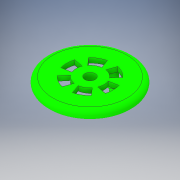
# Autodesk Inventor part: train wheel.
Saved by Autodesk Inventor 2017 (Build 210142000, 142)
## iProperties
Created: 2017-04-27
Part Number: train wheel.
Material: Generic
Document SubType Name: Modeling
Designer: 167898
Density: 1 g/cm^3
Appearance: Default
Author: 167898
Autodesk Inventor part; units mm, degrees
ref_plane "YZ Plane" through (0, 0, 0) normal (1, 0, 0) x (0, 1, 0)
ref_plane "XZ Plane" through (0, 0, 0) normal (0, 1, 0) x (-1, 0, 0)
ref_plane "XY Plane" through (0, 0, 0) normal (0, 0, 1) x (1, 0, 0)
sketch "Sketch1" plane through (0, 0, 0) normal (1, 0, 0) x (0, 1, 0)
  line L0 (0, 0) -> (6.3666, 0)
  line L1 (6.3666, 0) -> (6.3666, 25.3503)
  arc A0 (6.3666, 25.3503) -> (0, 25.3503) centre (3.1833, 25.5057) ccw
  line L2 (0, 25.3503) -> (0, 19.0141)
  line L3 (0, 19.0141) -> (3.1833, 19.0141)
  line L4 (3.1833, 19.0141) -> (3.1833, 6.3263)
  line L5 (3.1833, 6.3263) -> (0, 6.3263)
  line L6 (0, 6.3263) -> (0, 0)
  constraints: 14 end point, 5 perpendicular, 2 point on circle, 1 centre point, 1 horizontal, 1 point on line, 1 vertical
revolve "Revolution1" add sketch "Sketch1" angle 360 about axis through (0, 0, 0) along (0, 1, 0)
fillet "Fillet1" radius 1.5875 4 edges at (0, 0, -19.0141) (0, 3.1833, -19.0141) (0, 0, -6.3263) (0, 3.1833, -6.3263)
sketch "Sketch2" plane through (0, 0, 0) normal (0, -1, 0) x (1, 0, 0)
  point P0 (0, 0)
hole "Hole1" at (0, 0, 0) direction (0, 1, 0) diameter 7.112 end through all
sketch "Sketch3" plane through (0, 6.3666, 0) normal (0, 1, 0) x (1, 0, 0)
  circle A0 centre (0, 0) radius 3.556 projected
  circle A1 centre (0, 0) radius 9.525
  circle A2 centre (0, 0) radius 15.875
  line L0 (15.1682, 4.6843) -> (8.8363, 3.556)
  line L1 (15.1682, -4.6843) -> (8.8363, -3.556)
  line L2 (-3.556, 15.4716) -> (-2.4397, 9.2072)
  line L3 (3.556, 15.4716) -> (2.4397, 9.2072)
  dimension "d9" = 19.05
  dimension "d10" = 31.75
  constraints: 8 end point, 8 point on circle, 2 centre point, 2 coincident
  measures "d9" diameter of A1
  measures "d10" diameter of A2
extrude "Extrusion1" cut sketch "Sketch3" against normal blind 11.9126 contours A1 L0 A2 L1
pattern_circular "Circular Pattern1" count 6 over 360 about axis through (0, 81.4055, 0) along (0, -1, 0) of "Extrusion1"
sketch "Sketch4" plane through (0, 3.1833, 0) normal (0, -1, 0) x (1, 0, 0)
  circle A0 centre (0, -15.282) radius 3.175
  point P0 (0, 0)
  dimension "d16" = 6.35
  constraints: 1 centre point
  measures "d16" diameter of A0
extrude "Extrusion2" add sketch "Sketch4" along normal blind 9.525
sketch "Sketch5" plane through (0, -6.3417, -15.282) normal (0, -1, 0) x (1, 0, 0)
  circle A0 centre (0, 0) radius 1.5875
  point P0 (0, 15.282)
  dimension "d19" = 3.175
  constraints: 1 centre point
  measures "d19" diameter of A0
extrude "Extrusion3" add sketch "Sketch5" along normal blind 3.175
sketch "Sketch6" plane through (0, -9.5167, -15.282) normal (0, -1, 0) x (1, 0, 0)
  point P0 (0, 15.282)
  point P1 (0, 0)
hole "Hole2" at (0, -9.5167, -15.282) direction (0, 1, 0) diameter 2.032 depth 1.5875 tip angle 118
body "Solid1"
